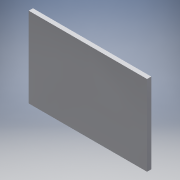
# Autodesk Inventor part: wall 1
Saved by Autodesk Inventor 2016 (Build 200138000, 138)
## iProperties
Created: 2017-03-30
Part Number: wall 1
Material: Aluminum 6061
Document SubType Name: Modeling
Designer: Ethan
Density: 2.7 g/cm^3
Appearance: Aluminum - Flat
Mass: 387.144 g
Surface Area: 490.322 cm^2
Volume: 143.387 cm^3
Author: Ethan
Autodesk Inventor part; units mm, degrees
ref_plane "YZ Plane" through (0, 0, 0) normal (1, 0, 0) x (0, 1, 0)
ref_plane "XZ Plane" through (0, 0, 0) normal (0, 1, 0) x (-1, 0, 0)
ref_plane "XY Plane" through (0, 0, 0) normal (0, 0, 1) x (1, 0, 0)
sketch "Sketch1" plane through (0, 0, 0) normal (0, 0, 1) x (1, 0, 0)
  line L0 (0, 0) -> (177.8, 0)
  line L1 (177.8, 0) -> (177.8, 120.65)
  line L2 (177.8, 120.65) -> (0, 120.65)
  line L3 (0, 120.65) -> (0, 0)
  dimension "d0" = 177.8
  dimension "d1" = 120.65
  constraints: 8 end point, 2 parallel, 1 horizontal, 1 perpendicular
  measures "d0" distance of L1.end L2.end
  measures "d1" distance of L2.end L0.start
extrude "Extrusion1" add sketch "Sketch1" along normal blind 6.35
body "Solid1"
